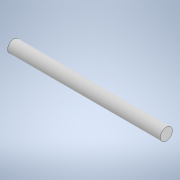
# Autodesk Inventor part: walek
Saved by Autodesk Inventor 2020 (Build 240168000, 168)
## iProperties
Created: 2020-03-28
Part Number: walek
Material: Ogólny
Document SubType Name: Modeling
Designer: niedz
Density: 1 g/cm^3
Appearance: Domyślna
Author: niedz
Autodesk Inventor part; units mm, degrees
ref_plane "YZ Plane" through (0, 0, 0) normal (1, 0, 0) x (0, 1, 0)
ref_plane "XZ Plane" through (0, 0, 0) normal (0, 1, 0) x (-1, 0, 0)
ref_plane "XY Plane" through (0, 0, 0) normal (0, 0, 1) x (1, 0, 0)
sketch "Szkic1" plane through (0, 0, 0) normal (1, 0, 0) x (0, 1, 0)
  circle A0 centre (0, 0) radius 1.5
  dimension "d1" = 3
  constraints: 1 centre point, 1 coincident
  measures "d1" diameter of A0
extrude "Wyciągnięcie proste2" add sketch "Szkic1" along normal blind 37.7
